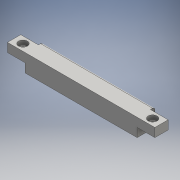
# Autodesk Inventor part: beam10cm
Saved by Autodesk Inventor 2016 (Build 200138000, 138)
## iProperties
Created: 2015-11-25
Part Number: beam10cm
Material: Generic
Document SubType Name: Modeling
Designer: hesaon
Density: 1 g/cm^3
Appearance: Default
Author: hesaon
Autodesk Inventor part; units mm, degrees
ref_plane "YZ Plane" through (0, 0, 0) normal (1, 0, 0) x (0, 1, 0)
ref_plane "XZ Plane" through (0, 0, 0) normal (0, 1, 0) x (-1, 0, 0)
ref_plane "XY Plane" through (0, 0, 0) normal (0, 0, 1) x (1, 0, 0)
sketch "Sketch1" plane through (0, 0, 0) normal (0, 0, 1) x (1, 0, 0)
  line L0 (0, 0) -> (100, 0)
  line L1 (100, 0) -> (100, 9)
  line L2 (88, 12) -> (12, 12)
  line L3 (0, 9) -> (0, 0)
  line L4 (12, 12) -> (12, 9)
  line L5 (12, 9) -> (0, 9)
  line L6 (88, 12) -> (88, 9)
  line L7 (88, 9) -> (100, 9)
  dimension "d6" = 100
  dimension "d7" = 3
  dimension "d8" = 3
  dimension "d9" = 12
  dimension "d10" = 12
  dimension "d11" = 9
  dimension "d12" = 9
  dimension "d13" = 12
  constraints: 16 end point, 2 parallel, 1 horizontal, 1 perpendicular
  measures "d6" distance of L0.end L0.start
  measures "d7" distance of L2.end L4.end
  measures "d8" distance of L6.end L2.start
  measures "d9" distance between parallel lines of L4 L3
  measures "d10" distance between parallel lines of L1 L6
  measures "d11" distance of L3.start L0.start
  measures "d12" distance of L1.end L0.end
  measures "d13" distance from line of L0 L2.end
extrude "Extrusion1" add sketch "Sketch1" along normal blind 6
sketch "Sketch2" plane through (0, 0, 0) normal (0, 0, -1) x (-1, 0, 0)
  line L0 (-88, 12) -> (-12, 12) projected
  line L1 (0, 0) -> (-100, 0) projected
  line L2 (-88, 12) -> (-12, 12)
  line L3 (-12, 12) -> (-12, 0)
  line L4 (-12, 0) -> (-88, 0)
  line L5 (-88, 0) -> (-88, 12)
  constraints: 8 end point, 2 parallel, 1 horizontal, 1 perpendicular, 1 point on line
extrude "Extrusion2" add sketch "Sketch2" along normal blind 6
sketch "Sketch3" plane through (0, 0, 0) normal (0, 0, -1) x (-1, 0, 0)
  circle A0 centre (-6, 4.5) radius 1.725
  line L0 (-12, 9) -> (0, 9) projected
  line L1 (0, 9) -> (0, 0) projected
  circle A1 centre (-94, 4.5) radius 1.725
  line L2 (-88, 0) -> (-100, 0) projected
  line L3 (-100, 0) -> (-100, 9) projected
  dimension "d18" = 3.45
  dimension "d19" = 4.5
  dimension "d20" = 6
  dimension "d21" = 3.45
  dimension "d22" = 4.5
  dimension "d23" = 6
  constraints: 2 centre point
  measures "d18" diameter of A0
  measures "d19" distance from line of L0 A0.centre
  measures "d20" distance from line of L1 A0.centre
  measures "d21" diameter of A1
  measures "d22" distance from line of L2 A1.centre
  measures "d23" distance from line of L3 A1.centre
extrude "Extrusion3" cut sketch "Sketch3" against normal blind 3
sketch "Sketch4" plane through (0, 0, 6) normal (0, 0, 1) x (1, 0, 0)
  circle A0 centre (6, 4.5) radius 3
  line L0 (12, 9) -> (0, 9) projected
  line L1 (0, 9) -> (0, 0) projected
  circle A1 centre (94, 4.5) radius 1.725 projected
  circle A2 centre (94, 4.5) radius 3
  dimension "d26" = 6
  dimension "d27" = 4.5
  dimension "d28" = 6
  dimension "d29" = 6
  constraints: 2 centre point, 1 coincident
  measures "d26" diameter of A0
  measures "d27" distance from line of L0 A0.centre
  measures "d28" distance from line of L1 A0.centre
  measures "d29" diameter of A2
extrude "Extrusion4" cut sketch "Sketch4" against normal blind 3 contours A0 | A1 | A2
fillet "Fillet1" radius 1.5 2 edges at (50, 12, 6) (50, 12, -6)
equation "\"d8\" = d7"
equation "\"d10\" = d9"
equation "\"d12\" = d11"
body "Solid1"
